clamp square nuts_v4 (Autodesk Fusion 360 design; units mm, degrees)
Autodesk Fusion 360 part; units mm, degrees
sketch "Sketch1" plane through (0, 0, 0) normal (0, 0, 1) x (1, 0, 0) in component "link"
  line L0 (0, 0) -> (14, 0)
  line L1 (14, 0) -> (14, -14)
  line L2 (14, -14) -> (0, -14)
  line L3 (0, -14) -> (0, 0)
  circle A0 centre (7, -7) radius 5
  circle A1 centre (7, -7) radius 1.95
  dimension "d68" = 14
  dimension "d69" = 10
  dimension "d70" = 7
  dimension "d72" = 3.9
  dimension "d105" = 14
  dimension "d106" = 7
  constraint horizontal L0
  constraint vertical L1
  constraint horizontal L2
  constraint vertical L3
  constraint coincident L0.start L3.end
  constraint concentric A0 A1
  measures "d68" distance of L0.start L2.end
  measures "d69" diameter of A0
  measures "d70" distance of L0 A0.centre
  measures "d72" diameter of A1
  measures "d105" distance of L1.end L2.end
  measures "d106" distance of L3 A0.centre
extrude "Extrude3" add sketch "Sketch1" along normal blind 6.5 contours L0 L1 L2 L3 | A0 | A1 in component "link"
extrude "Extrude4" cut sketch "Sketch1" along normal up to surface (6.5 mm away) contours A1 in component "link"
ref_plane "WorkPlane1" through (7, -7, 3.25) normal (1, 0, 0) x (0, 1, 0)
sketch "Sketch3" plane through (7, -7, 3.5) normal (1, 0, 0) x (0, 1, 0) in component "link"
  line L0 (0, 0) -> (14, 0) construction
  line L1 (14, 0) -> (14, 7) construction
  line L2 (14, 7) -> (0, 7)
  line L3 (0, 7) -> (0, 0) construction
  line L4 (5.5, 3.0262) -> (0, -0.9738)
  line L5 (0, -0.9738) -> (0, 3.0262)
  line L6 (0, 3.0262) -> (5.5, 3.0262)
  point P0 (7, 0)
  dimension "d109" = 5.5
  dimension "d110" = 4
  constraint coincident L3 L4.end
  constraint perpendicular L3 L6
  constraint coincident L3 L5.end
  measures "d109" horizontal distance of L0.start L4.start
  measures "d110" distance of L5.end L4.end
revolve "Revolve1" cut sketch "Sketch3" angle 360 about axis through (7, -7, 10.5) along (0, 0, -1) in component "link"
fillet "Fillet2" radius 1 4 edges at (0, -14, 3.25) (0, 0, 3.25) (14, -14, 3.25) (14, 0, 3.25) in component "link"
component "link" placed x (1, 0, 0) y (0, 1, 0) z (0, 0, 1) at (0, 0, 0)
equation "ballJointHoleDim = 22.3 mm"
equation "tubeThickness = 2 mm"
equation "stockThickness = 9.6 mm"
equation "baseHeight = 5.5 mm"
equation "screwsCenterDistance = 32 mm"
equation "baseLength = 42 mm"
equation "ballJointBottomFromGround = 2 mm"
equation "screwHoleDiam = 3.5 mm"
equation "screwHeadHoleDiam = 6.3 mm"
equation "screwHeadHeight = 2 mm"
equation "ballJointHeight = 7 mm"
equation "linkStockHeight = 12.8 mm"
equation "linkWidth = 9.4 mm"
equation "linkHoleCenterDistance = 41 mm"
equation "linkBallJoinInsertDiam = 8.1 mm"
equation "linkBallInsertHeight = 6.8 mm"
equation "linkClearanceHeigt = 1 mm"
equation "toolDiameter = 2 mm"
